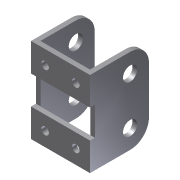
# Autodesk Inventor part: JointC3_2nd
Saved by Autodesk Inventor 2011 SP1 (Build 150282100, 282)
## iProperties
Created: 2013-02-06
Part Number: JointC3_2nd
Document SubType Name: Modeling
Designer: arihon
Density: 1 g/cm^3
Author: arihon
Autodesk Inventor part; units mm, degrees
ref_plane "YZ Plane" through (0, 0, 0) normal (1, 0, 0) x (0, 1, 0)
ref_plane "XZ Plane" through (0, 0, 0) normal (0, 1, 0) x (-1, 0, 0)
ref_plane "XY Plane" through (0, 0, 0) normal (0, 0, 1) x (1, 0, 0)
sketch "スケッチ1" plane through (0, 0, 0) normal (0, 0, 1) x (1, 0, 0)
  line L0 (-12.5, 25) -> (12.5, 25)
  line L1 (12.5, 25) -> (12.5, 0)
  line L2 (12.5, 0) -> (-12.5, 0)
  line L3 (-12.5, 0) -> (-12.5, 25)
  line L4 (-10.5, 25) -> (10.5, 25)
  line L5 (10.5, 25) -> (10.5, 2)
  line L6 (10.5, 2) -> (-10.5, 2)
  line L7 (-10.5, 2) -> (-10.5, 25)
  point P0 (0, 0)
  dimension "d0" = 25
  dimension "d1" = 25
  dimension "d2" = 0
  dimension "d3" = 12.5
  dimension "d4" = 2
  dimension "d5" = 2
  dimension "d6" = 2
  constraints: 16 end point, 4 parallel, 2 horizontal, 2 perpendicular, 1 point on line
  measures "d0" distance of L0.start L0.end
  measures "d1" distance of L0.end L1.end
  measures "d2" distance from line of L2 point (0, 0)
  measures "d3" distance from line of point (0, 0) L1
  measures "d4" distance between parallel lines of L3 L7
  measures "d5" distance between parallel lines of L1 L5
  measures "d6" distance between parallel lines of L2 L6
extrude "押し出し1" add sketch "スケッチ1" along normal blind 36 contours L0 L7 L6 L5 L1 L2 L3
sketch "スケッチ2" plane through (12.5, 0, 0) normal (1, 0, 0) x (0, 0, -1)
  line L0 (-36, 25) -> (-36, 0) projected
  line L1 (0, 25) -> (-36, 25) projected
  point P0 (-28, 17)
  point P1 (-8, 17)
  dimension "d9" = 20
  dimension "d10" = 8
  dimension "d11" = 8
  dimension "d12" = 8
  measures "d9" distance of point (-8, 17) point (-28, 17)
  measures "d10" distance from line of L0 point (-28, 17)
  measures "d11" distance from line of point (-28, 17) L1
  measures "d12" distance from line of point (-8, 17) L1
hole "Hole1" at (12.5, 17, 28) at (12.5, 17, 8) direction (-1, 0, 0) diameter 6 end through all
fillet "フィレット1" radius 8 4 edges at (11.5, 25, 36) (-11.5, 25, 36) (-11.5, 25, 0) (11.5, 25, 0)
sketch "スケッチ3" plane through (-10.5, 2, 36) normal (0, 1, 0) x (1, 0, 0)
  line L0 (21, 0) -> (0, 0) projected
  line L1 (21, 36) -> (21, 0) projected
  line L2 (0, 36) -> (21, 36) projected
  line L3 (0, 36) -> (0, 0) projected
  point P0 (10.5, 36)
  point P1 (4, 30)
  point P2 (17, 30)
  point P3 (17, 6)
  point P4 (4, 6)
  dimension "d21" = 6
  dimension "d22" = 4
  dimension "d23" = 6
  dimension "d24" = 4
  dimension "d25" = 4
  dimension "d26" = 6
  dimension "d27" = 6
  dimension "d28" = 4
  measures "d21" distance from line of L2 point (4, 30)
  measures "d22" distance from line of L3 point (4, 30)
  measures "d23" distance from line of L2 point (17, 30)
  measures "d24" distance from line of L1 point (17, 30)
  measures "d25" distance from line of L3 point (4, 6)
  measures "d26" distance from line of L0 point (4, 6)
  measures "d27" distance from line of L0 point (17, 6)
  measures "d28" distance from line of L1 point (17, 6)
hole "Hole2" at (-6.5, 2, 6) at (6.5, 2, 6) at (6.5, 2, 30) at (-6.5, 2, 30) direction (0, -1, 0) diameter 3.2 end through all
sketch "スケッチ4" plane through (-12.5, 0, 0) normal (0, -1, 0) x (1, 0, 0)
  line L0 (0, 0) -> (0, 36) projected
  line L1 (25, 0) -> (25, 36) projected
  line L2 (25, 18) -> (0, 18)
  line L3 (0, 24.05) -> (25, 24.05)
  line L4 (25, 24.05) -> (25, 11.95)
  line L5 (25, 11.95) -> (0, 11.95)
  line L6 (0, 11.95) -> (0, 24.05)
  point P0 (12.5, 0)
  dimension "d36" = 12.1
  dimension "d37" = 12.1
  constraints: 10 end point, 2 midpoint, 2 parallel, 2 point on line, 1 horizontal, 1 perpendicular
  measures "d36" distance between parallel lines of L5 L3
  measures "d37" diameter of L5 L2
extrude "押し出し2" cut sketch "スケッチ4" against normal blind 2.1
equation "\"d1\" = d0"
equation "\"d3\" = 0.5 * d0"
equation "\"d5\" = d4"
equation "\"d6\" = d4"
equation "\"d10\" = d11"
equation "\"d12\" = d11"
equation "\"d23\" = d21"
equation "\"d24\" = d22"
equation "\"d25\" = d22"
equation "\"d26\" = d21"
equation "\"d27\" = d21"
equation "\"d28\" = d22"
equation "\"d37\" = d36"
